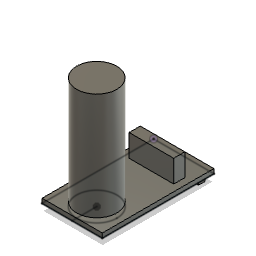
nixie_adapter v2 (Autodesk Fusion 360 design; units mm, degrees)
Autodesk Fusion 360 part; units mm, degrees
sketch "Skizze1" plane through (0, 0, 0) normal (0, 1, 0) x (1, 0, 0)
  line L0 (0, 0) -> (27, 0)
  line L1 (27, 0) -> (27, -50)
  line L2 (27, -50) -> (0, -50)
  line L3 (0, -50) -> (0, 0)
  line L4 (13.5, -50) -> (13.5, -39)
  circle A0 centre (13.5, -39) radius 9
  dimension "d1" = 50
  dimension "d2" = 27
  dimension "d3" = 11
  dimension "d4" = 18
  constraint horizontal L0
  constraint vertical L1
  constraint horizontal L2
  constraint vertical L3
  constraint coincident L0.start L3.end
  constraint midpoint L2 L4.start
  constraint perpendicular L2 L4
  constraint coincident L4.end A0.centre
  measures "d1" distance of L0.start L2.end
  measures "d2" distance of L0.start L0.end
  measures "d3" distance of L4.start L4.end
  measures "d4" diameter of A0
extrude "Extrusion1" add sketch "Skizze1" along normal blind 50 contours A0 makes body 1
extrude "Extrusion2" add sketch "Skizze1" along normal blind 2 bodies 1
sketch "Skizze2" plane through (0, 2, 0) normal (0, 1, 0) x (-1, 0, 0)
  circle A0 centre (-13.5, 39) radius 9
  line L0 (0, 50) -> (-27, 50)
  line L1 (-27, 50) -> (-27, 0)
  line L2 (-27, 0) -> (0, 0)
  line L3 (0, 0) -> (0, 50)
  line L4 (0, 0) -> (-4, 0)
  line L5 (-4, 0) -> (-4, 10)
  line L6 (-4, 10) -> (0, 10)
  line L7 (0, 10) -> (0, 0)
  line L8 (-4, 10) -> (-24, 10)
  line L9 (-24, 10) -> (-24, 15)
  line L10 (-24, 15) -> (-4, 15)
  line L11 (-4, 15) -> (-4, 10)
  dimension "d9" = 10
  dimension "d10" = 4
  dimension "d11" = 20
  dimension "d12" = 5
  constraint horizontal L4
  constraint vertical L5
  constraint horizontal L6
  constraint vertical L7
  constraint coincident L2.end L3.start
  constraint horizontal L8
  constraint vertical L9
  constraint horizontal L10
  constraint vertical L11
  measures "d9" distance of L2.end L6.end
  measures "d10" distance of L2.end L4.end
  measures "d11" distance of L5.end L8.end
  measures "d12" distance of L5.end L10.end
extrude "Extrusion3" add sketch "Skizze2" along normal blind 10 contours L8 L9 L10 L11 bodies 1
sketch "Skizze3" plane through (0, 2, 0) normal (0, 1, 0) x (-1, 0, 0)
  line L0 (-4, 15) -> (-4, 10)
  line L1 (-4, 10) -> (-24, 10)
  line L2 (-24, 10) -> (-24, 15)
  line L3 (-24, 15) -> (-4, 15)
  circle A0 centre (-13.5, 39) radius 9
  line L4 (0, 50) -> (-27, 50)
  line L5 (-27, 50) -> (-27, 0)
  line L6 (-27, 0) -> (0, 0)
  line L7 (0, 0) -> (0, 50)
  line L8 (-5, 5) -> (-25, 5)
  line L9 (-25, 5) -> (-25, 2)
  line L10 (-25, 2) -> (-5, 2)
  line L11 (-5, 2) -> (-5, 5)
  dimension "d15" = 20
  dimension "d16" = 3
  constraint horizontal L8
  constraint vertical L9
  constraint horizontal L10
  constraint vertical L11
  measures "d15" distance of L8.start L8.end
  measures "d16" distance of L8.start L10.end
extrude "Extrusion4" add sketch "Skizze3" against normal blind 5 contours L8 L9 L10 L11 bodies 1
copy_body "Körper->Berechn1" bodies 1 removing the originals makes body 2 in component "nixie_modul"
component "nixie_modul" placed x (1, 0, 0) y (0, 1, 0) z (0, 0, 1) at (0, 0, 0)
